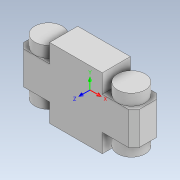
# Autodesk Inventor part: body_inventor
Saved by Autodesk Inventor 2020 (Build 240168000, 168)
## iProperties
Created: 2021-01-07
Part Number: body_inventor
Material: Generic
Document SubType Name: Modeling
Designer: DELL
Density: 1 g/cm^3
Appearance: Default
Author: DELL
Autodesk Inventor part; units mm, degrees
ref_plane "YZ Plane" through (0, 0, 0) normal (1, 0, 0) x (0, 1, 0)
ref_plane "XZ Plane" through (0, 0, 0) normal (0, 1, 0) x (-1, 0, 0)
ref_plane "XY Plane" through (0, 0, 0) normal (0, 0, 1) x (1, 0, 0)
sketch "Sketch4" plane through (0, 0, 0) normal (0, 0, 1) x (1, 0, 0)
  line L0 (75, -100) -> (-75, -100)
  line L1 (-75, -100) -> (-75, 100)
  line L2 (-75, 100) -> (75, 100)
  line L3 (75, 100) -> (75, -100)
  line L4 (75, -100) -> (-75, 100) construction
  line L5 (-75, -100) -> (75, 100) construction
  line L6 (165, -47) -> (-165, -47)
  line L7 (-165, -47) -> (-165, 47)
  line L8 (-165, 47) -> (165, 47)
  line L9 (165, 47) -> (165, -47)
  line L10 (165, -47) -> (-165, 47) construction
  line L11 (-165, -47) -> (165, 47) construction
  point P0 (0, 0)
  point P1 (0, 0)
  point P2 (0, 0)
  point P3 (75, 47)
  point P4 (-75, 47)
  point P5 (-75, -47)
  point P6 (75, -47)
  dimension "d17" = 94
  dimension "d18" = 330
  dimension "d19" = 150
  dimension "d20" = 200
  constraints: 24 end point, 5 midpoint, 4 parallel, 2 horizontal, 2 perpendicular, 1 coincident
  measures "d17" distance of L8.end L6.start
  measures "d18" distance of L6.start L6.end
  measures "d19" distance of L0.start L0.end
  measures "d20" distance of L2.end L0.start
extrude "Extrusion4" add sketch "Sketch4" along normal mid plane 80
sketch "Sketch5" plane through (0, 0, 0) normal (0, 1, 0) x (-1, 0, 0)
  circle A0 centre (-118, 0) radius 39.5
  circle A1 centre (118, 0) radius 39.5
  line L0 (75, 40) -> (-75, 40) construction
  line L1 (0, 40) -> (0, -40) construction
  line L2 (-75, -40) -> (75, -40) construction
  line L3 (-165, -40) -> (-165, 40) construction
  line L4 (-165, 0) -> (165, 0) construction
  line L5 (165, 40) -> (165, -40) construction
  circle A2 centre (-118, 0) radius 31.5
  circle A3 centre (118, 0) radius 31.5
  line L6 (-150, 40) -> (-165, 25)
  line L7 (-165, -25) -> (-150, -40)
  line L8 (-165, -40) -> (-75, -40) projected
  line L9 (165, 40) -> (75, 40) projected
  line L10 (150, 40) -> (165, 25)
  line L11 (165, -25) -> (150, -40)
  line L12 (-75, 40) -> (-165, 40) projected
  line L13 (75, -40) -> (165, -40) projected
  line L14 (-165, 40) -> (-165, -40)
  line L15 (165, 40) -> (165, -40)
  point P0 (0, 0)
  dimension "d23" = 79
  dimension "d24" = 236
  dimension "d39" = 63
  dimension "d42" = 15
  dimension "d43" = 45
  constraints: 16 end point, 9 point on line, 5 perpendicular, 4 centre point, 4 midpoint, 3 equal length, 2 coincident, 2 equal radius, 1 symmetric about line
  measures "d23" diameter of A0
  measures "d24" distance of A1.centre A0.centre
  measures "d39" diameter of A2
  measures "d42" distance of L3.end L6.end
  measures "d43" angle of L6 L3
extrude "Extrusion5" add sketch "Sketch5" against normal blind 32 from surface at -47 contours A0 | A1 | A2 | A3
sketch "Sketch6" plane through (0, 0, 0) normal (0, 0, 1) x (1, 0, 0)
  line L0 (142, 25) -> (-142, 25)
  line L1 (-142, 25) -> (-142, -25)
  line L2 (-142, -25) -> (142, -25)
  line L3 (142, -25) -> (142, 25)
  line L4 (142, 25) -> (-142, -25) construction
  line L5 (-142, 25) -> (142, -25) construction
  line L6 (-65, 90) -> (65, 90)
  line L7 (65, 90) -> (65, -90)
  line L8 (65, -90) -> (-65, -90)
  line L9 (-65, -90) -> (-65, 90)
  line L10 (-65, 90) -> (65, -90) construction
  line L11 (65, 90) -> (-65, -90) construction
  line L12 (75, -100) -> (-75, -100) projected
  line L13 (-75, 47) -> (-75, 100) projected
  line L14 (-165, -47) -> (-165, 47) projected
  line L15 (-75, -47) -> (-165, -47) projected
  point P0 (0, 0)
  point P1 (-65, -25)
  point P2 (65, -25)
  point P3 (65, 25)
  point P4 (-65, 25)
  dimension "d27" = 10
  dimension "d28" = 10
  dimension "d29" = 23
  dimension "d30" = 22
  constraints: 24 end point, 4 midpoint, 4 parallel, 2 horizontal, 2 perpendicular
  measures "d27" distance between parallel lines of L12 L8
  measures "d28" distance between parallel lines of L13 L9
  measures "d29" distance between parallel lines of L14 L1
  measures "d30" distance between parallel lines of L15 L2
extrude "Extrusion6" cut sketch "Sketch6" along normal mid plane 60
extrude "Extrusion8" cut sketch "Sketch5" against normal through all both and the other way through all contours L6 L14 L12 | L7 L8 L14 | L15 L10 L9 | L15 L13 L11
mirror "Mirror1" about plane through (0, 0, 0) normal (0, 1, 0) of "Extrusion5"
body "Solid1"
body "Solid2"
